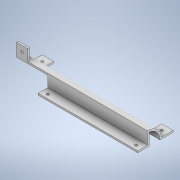
# Autodesk Inventor part: CableCoverForFrameHigher
Saved by Autodesk Inventor 2021.3 (Build 253353000, 353)
## iProperties
Created: 2021-05-28
Part Number: CableCoverForFrameHigher
Material: 一般
Document SubType Name: Modeling
Designer: gisen
Density: 1 g/cm^3
Appearance: 既定
Author: gisen
Autodesk Inventor part; units mm, degrees
sketch "スケッチ1" plane through (0, 0, 0) normal (0, 1, 0) x (-1, 0, 0)
  line L0 (0, -22) -> (230, -22)
  line L1 (230, -22) -> (230, -25)
  line L2 (230, -25) -> (0, -25)
  line L3 (0, -25) -> (0, -22)
  line L4 (276, 0) -> (-46, 0) projected
  point P0 (0, 0)
  dimension "d0" = 3
  dimension "d1" = 230
  dimension "d2" = 25
  constraints: 8 end point, 2 parallel, 1 horizontal, 1 perpendicular
  measures "d0" distance of L2.end L0.start
  measures "d1" distance of L1.end L2.end
  measures "d2" distance of point (0, 0) L2.end
revolve "回転1" add sketch "スケッチ1" angle 90 about axis through (-10, 0, 0) along (1, 0, 0)
sketch "スケッチ2" plane through (-230, 25, 0) normal (0, 0, 1) x (1, 0, 0)
  line L0 (230, 0) -> (0, 0) projected
  line L1 (0, 0) -> (0, -3) projected
  line L2 (0, -3) -> (230, -3) projected
  line L3 (230, -3) -> (230, 0) projected
  line L4 (230, 0) -> (0, 0) projected
  line L5 (0, 0) -> (20, 0)
  line L6 (20, 0) -> (20, 20)
  line L7 (20, 20) -> (0, 20)
  line L8 (0, 20) -> (0, 0)
  line L9 (115, 0) -> (115, -3)
  line L10 (0, -3) -> (230, -3) projected
  line L11 (20, 0) -> (20, -3)
  circle A0 centre (10, 10) radius 2.25
  point P0 (230, -25)
  point P1 (20, 0)
  point P2 (20, -3)
  point P3 (20, 0)
  dimension "d4" = 20
  dimension "d5" = 20
  dimension "d8" = 4.5
  constraints: 12 end point, 2 midpoint, 2 parallel, 2 perpendicular, 1 centre point, 1 horizontal, 1 point on line
  measures "d4" distance of L7.end L0.end
  measures "d5" distance of L6.end L7.end
  measures "d8" diameter of A0
extrude "押し出し1" add sketch "スケッチ2" against normal blind 3 contours L11 L2 L1 L0 | L0 L8 L7 L6
ref_plane "作業平面1" through (-115, 0, -25) normal (-1, 0, 0) x (0, 0, 1)
mirror "ミラー1" about plane through (-115, 0, -25) normal (-1, 0, 0) of "押し出し1"
ref_plane "作業平面2" through (-230, 0, 0) normal (0, 0.7071068, 0.7071068) x (-1, 0, 0)
mirror "ミラー2" about plane through (-230, 0, 0) normal (0, 0.7071068, 0.7071068) of "ミラー1", "押し出し1"
ref_plane "作業平面3" through (-20, 22, 0) normal (0, 1, 0) x (1, 0, 0)
sketch "スケッチ4" plane through (-20, 22, 0) normal (0, 1, 0) x (1, 0, 0)
  line L0 (0, 0) -> (20, 0) projected
  line L1 (20, 0) -> (20, 3) projected
  line L2 (20, 3) -> (0, 3) projected
  line L3 (0, 0) -> (0, 3) projected
  line L4 (20, 0) -> (0, 0)
  line L5 (0, 0) -> (-155, 0)
  line L6 (-155, 0) -> (-155, 3)
  line L7 (-155, 3) -> (0, 3)
  line L8 (0, 3) -> (0, 0)
  line L9 (-210, 0) -> (-210, 22) projected
  dimension "d22" = 55
  constraints: 10 end point, 2 horizontal, 2 parallel, 1 perpendicular
  measures "d22" distance between parallel lines of L9 L6
extrude "押し出し3" add sketch "スケッチ4" against normal up to surface (22 mm away)
sketch "スケッチ5" plane through (-230, 45, 0) normal (0, 0, 1) x (1, 0, 0)
  line L0 (230, -45) -> (55, -45) projected
  line L1 (230, -42) -> (210, -42) projected
  line L2 (230, 0) -> (230, -45) projected
  line L3 (210, -42) -> (55, -42)
  line L4 (55, -23.2055) -> (55, -45) projected
  line L5 (55, -23) -> (55, -45) projected
  constraints: 2 end point, 1 horizontal, 1 point on line
extrude "押し出し4" add sketch "スケッチ5" along normal blind 17
sketch "スケッチ7" plane through (-175, 3, 0) normal (0, 1, 0) x (1, 0, 0)
  circle A0 centre (165, 35) radius 2.25 projected
  circle A1 centre (165, -10) radius 2.25
  line L0 (0, 0) -> (175, 0) projected
  line L1 (175, 0) -> (175, -17) projected
  circle A2 centre (10, -10) radius 2.25
  line L2 (0, 0) -> (0, -17) projected
  dimension "d23" = 4.5
  dimension "d24" = 10
  dimension "d25" = 10
  dimension "d26" = 4.5
  dimension "d27" = 10
  dimension "d28" = 10
  constraints: 2 centre point
  measures "d23" diameter of A1
  measures "d24" distance from line of L0 A1.centre
  measures "d25" distance from line of L1 A1.centre
  measures "d26" diameter of A2
  measures "d27" distance from line of L2 A2.centre
  measures "d28" distance from line of L0 A2.centre
extrude "押し出し6" cut sketch "スケッチ7" against normal up to surface (3 mm away) contours A1 | A2
sketch "スケッチ8" plane through (0, 24.8193, -3) normal (1, 0, 0) x (0, 0, -1)
  arc A0 (19, -24.8193) -> (0, -3.0249) centre (-3, -24.8193) ccw projected
  line L0 (19, -24.8193) -> (42, -24.8193) projected
  line L1 (42, -24.8193) -> (42, -21.8193) projected
  line L2 (21.8193, -21.8193) -> (42, -21.8193) projected
  arc A1 (21.8193, -21.8193) -> (0, 0) centre (-3, -24.8193) ccw projected
  line L3 (0, 0) -> (0, 20.1807) projected
  line L4 (-3, 20.1807) -> (0, 20.1807) projected
  line L5 (-3, 20.1807) -> (-3, -21.8193) projected
  line L6 (-3, -21.8193) -> (-20, -21.8193) projected
  line L7 (-20, -24.8193) -> (-20, -21.8193) projected
  line L8 (0, -24.8193) -> (-20, -24.8193) projected
  line L9 (0, -3.0249) -> (0, -24.8193) projected
  line L10 (-3, 20.1807) -> (-3, -21.8193) projected
  arc A2 (0, 0) -> (-3, 0.1807) centre (-3, -24.8193) ccw
  point P0 (-3, -24.8193)
  point P1 (-3, 0.1807)
  constraints: 2 point on circle, 1 centre point, 1 coincident, 1 point on line
extrude "押し出し7" cut sketch "スケッチ8" against normal up to surface (20 mm away) contours A2 L5 L4 L3
